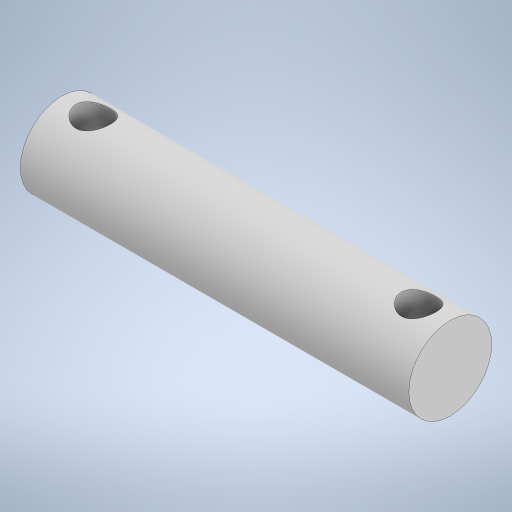
# Autodesk Inventor part: Wrist Pin
Saved by Autodesk Inventor 2023 (Build 270158000, 158)
## iProperties
Created: 2022-11-15
Part Number: Wrist Pin
Material: Generic
Document SubType Name: Modeling
Designer: tommy
Density: 1 g/cm^3
Appearance: Default
Author: tommy
Autodesk Inventor part; units mm, degrees
ref_plane "YZ Plane" through (0, 0, 0) normal (1, 0, 0) x (0, 1, 0)
ref_plane "XY Plane" through (0, 0, 0) normal (0, 0, 1) x (1, 0, 0)
sketch "Sketch1" plane through (0, 0, 0) normal (1, 0, 0) x (0, 1, 0)
  circle A0 centre (0, 0) radius 3.048
  dimension "d0" = 6.096
  constraints: 1 centre point, 1 coincident
  measures "d0" diameter of A0
extrude "Extrusion1" add sketch "Sketch1" along normal blind 28.575
ref_plane "Work Plane1" through (0, 4.7625, 0) normal (0, 1, 0) x (-1, 0, 0)
sketch "Sketch2" plane through (0, 4.7625, 0) normal (0, 1, 0) x (-1, 0, 0)
  line L0 (0, 0) -> (-28.575, 0)
  line L1 (-28.575, 3.048) -> (-28.575, -3.048) projected
  line L2 (-14.2875, 0) -> (-26.2509, 0)
  line L3 (-26.2509, 0) -> (-24.7932, 0)
  line L4 (-14.2875, 0) -> (-2.3241, 0)
  circle A0 centre (-26.2509, 0) radius 1.27
  circle A1 centre (-2.3241, 0) radius 1.27
  dimension "d4" = 11.9634
  dimension "d5" = 11.9634
  dimension "d6" = 2.54
  dimension "d9" = 2.54
  constraints: 8 end point, 3 point on line, 2 centre point, 2 coincident, 2 midpoint
  measures "d4" distance of L2.start L2.end
  measures "d5" distance of L2.start L4.end
  measures "d6" diameter of A1
  measures "d9" diameter of A0
extrude "Extrusion2" cut sketch "Sketch2" against normal blind 25.4
body "Solid1"
